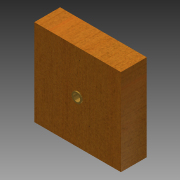
# Autodesk Inventor part: Door
Saved by Autodesk Inventor 2014 (Build 180170000, 170)
## iProperties
Created: 2014-03-19
Part Number: Door
Material: Generic
Document SubType Name: Modeling
Designer: Alex
Density: 1 g/cm^3
Appearance: Yellow Pine - Solid Stained Light Low Gloss
Author: Alex
Autodesk Inventor part; units mm, degrees
ref_plane "YZ Plane" through (0, 0, 0) normal (1, 0, 0) x (0, 1, 0)
ref_plane "XZ Plane" through (0, 0, 0) normal (0, 1, 0) x (-1, 0, 0)
ref_plane "XY Plane" through (0, 0, 0) normal (0, 0, 1) x (1, 0, 0)
sketch "Sketch1" plane through (0, 0, 0) normal (0, 0, 1) x (1, 0, 0)
  line L0 (0, 0) -> (152.4, 0)
  line L1 (152.4, 0) -> (152.4, 152.4)
  line L2 (152.4, 152.4) -> (0, 152.4)
  line L3 (0, 152.4) -> (0, 0)
  dimension "d0" = 152.4
  dimension "d1" = 152.4
  constraints: 8 end point, 2 parallel, 1 horizontal, 1 perpendicular
  measures "d0" distance of L2.end L0.start
  measures "d1" distance of L0.start L0.end
extrude "Extrusion1" add sketch "Sketch1" along normal blind 45.339
sketch "Sketch2" plane through (0, 0, 45.339) normal (0, 0, 1) x (1, 0, 0)
  line L0 (0, 0) -> (152.4, 0) projected
  line L1 (0, 152.4) -> (0, 0) projected
  circle A0 centre (76.2, 76.2) radius 6.35
  circle A1 centre (76.2, 76.2) radius 9.017
  dimension "d13" = 12.7
  dimension "d14" = 18.034
  dimension "d15" = 76.2
  dimension "d16" = 76.2
  constraints: 2 centre point, 1 coincident
  measures "d13" diameter of A0
  measures "d14" diameter of A1
  measures "d15" distance from line of L1 A0.centre
  measures "d16" distance from line of L0 A0.centre
extrude "Extrusion2" add sketch "Sketch2" along normal blind 1.905
hole "Hole2" at (76.2, 76.2, 45.339) direction (0, 0, -1) diameter 12.7 depth 18.415
hole "Hole3" at (76.2, 76.2, 26.924) direction (0, 0, -1) diameter 12.192 depth 7.747
hole "Hole4" at (76.2, 76.2, 19.177) direction (0, 0, -1) diameter 11.684 depth 0.508
body "Solid1"
